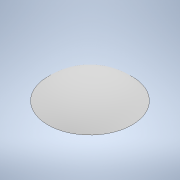
# Autodesk Inventor part: soczewka
Saved by Autodesk Inventor 2020 (Build 240168000, 168)
## iProperties
Created: 2019-12-30
Part Number: soczewka
Material: Ogólny
Document SubType Name: Modeling
Designer: macie
Density: 1 g/cm^3
Appearance: Domyślna
Author: macie
Autodesk Inventor part; units mm, degrees
ref_plane "YZ Plane" through (0, 0, 0) normal (1, 0, 0) x (0, 1, 0)
ref_plane "XZ Plane" through (0, 0, 0) normal (0, 1, 0) x (-1, 0, 0)
ref_plane "XY Plane" through (0, 0, 0) normal (0, 0, 1) x (1, 0, 0)
sketch "Szkic1" plane through (0, 0, 0) normal (0, 0, 1) x (1, 0, 0)
  line L0 (0, 0) -> (9.025, 0)
  line L1 (0, 0) -> (9.025, 0) construction
  line L2 (0, 0) -> (0, 4)
  arc A0 (9.025, 0) -> (0, 4) centre (0.0585, -8.0494) ccw
  dimension "d0" = 9.025
  dimension "d1" = 0
  dimension "d2" = 4
  constraints: 6 end point, 2 horizontal, 2 point on circle, 1 centre point, 1 collinear, 1 vertical
  measures "d0" distance of L0.start L0.end
  measures "d1" distance between parallel lines of L0 L1
  measures "d2" distance of L0.start L2.end
revolve "Obrót1" add sketch "Szkic1" angle 360 about axis through (0, 0, 0) along (0, 1, 0)
